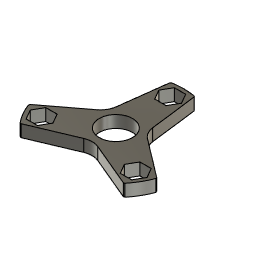
Fidget Spinner v0 (Autodesk Fusion 360 design; units mm, degrees)
Autodesk Fusion 360 part; units mm, degrees
sketch "Sketch1" plane through (0, 0, 0) normal (0, 0, 1) x (1, 0, 0)
  circle A0 centre (0, 0) radius 45
  circle A1 centre (0, 0) radius 11
  circle A2 centre (0, 0) radius 4
  circle A3 centre (0, 0) radius 13.5
  line L0 (7.5056, 36) -> (3.7528, 42.5)
  line L1 (3.7528, 42.5) -> (-3.7528, 42.5)
  line L2 (-3.7528, 42.5) -> (-7.5056, 36)
  line L3 (-7.5056, 36) -> (-3.7528, 29.5)
  line L4 (-3.7528, 29.5) -> (3.7528, 29.5)
  line L5 (3.7528, 29.5) -> (7.5056, 36)
  line L6 (0, 0) -> (0, 29.5) construction
  circle A4 centre (0, 36) radius 9 construction
  line L7 (-13.3941, 1.6875) -> (-8.0282, 44.2781)
  line L8 (8.0282, 44.2781) -> (13.3941, 1.6875)
  point P0 (0, 36)
  dimension "d1" = 90
  dimension "d2" = 22
  dimension "d3" = 8
  dimension "d4" = 2.5
  dimension "d5" = 6.5
  dimension "d6" = 29.5
  constraint coincident A0.centre A1.centre
  constraint concentric A1 A2
  constraint midpoint L4 L6.end
  constraint vertical L6
  constraint perpendicular L4 L6
  constraint coincident P0 A4.centre
  constraint tangent A0 A4
  constraint coincident A3 L7.start
  constraint coincident A0 L7.end
  constraint tangent A3 L7
  constraint tangent A4 L7
  constraint coincident A0 L8.start
  constraint coincident A3 L8.end
  constraint tangent A3 L8
  constraint tangent A4 L8
  measures "d1" diameter of A0
  measures "d2" diameter of A1
  measures "d3" diameter of A2
  measures "d4" distance of A1 A3
  measures "d5" distance of P0 L5
  measures "d6" distance of A0.centre L6.end
extrude "Extrude1" add sketch "Sketch1" along normal blind 8 contours A0 A3 L7 L8 | A3 picked at (0, 24.1667) makes body 1
pattern_circular "C-Pattern1" count 3 over 360 about axis through (0, 0, 1.75) along (0, 0, 1) of bodies 1 makes body 2 at (-20.0614, -11.8988, 0) makes body 3 at (20.3354, -11.4242, 0)
combine "Combine1" operation add target body 1 tool bodies 3 2
fillet "Fillet1" radius 12 3 edges at (12.6841, 7.3232, 4) (-12.6841, 7.3232, 4) (0, -14.6463, 4) on bodies 1
chamfer "Chamfer1" distance 0.5 angle 45 6 edges at (-8.0282, 44.2781, 4) (8.0282, 44.2781, 4) (42.36, -15.1864, 4) (-42.36, -15.1864, 4) (-34.3318, -29.0917, 4) (34.3318, -29.0917, 4) on bodies 1
